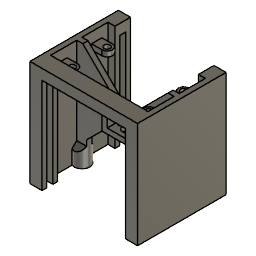
Pot_v21 (Autodesk Fusion 360 design; units mm, degrees)
Autodesk Fusion 360 part; units mm, degrees
sketch "Sketch1" plane through (0, 0, 0) normal (0, 0, 1) x (1, 0, 0)
  line L0 (0, -19.5) -> (-28, -19.5) construction
  line L1 (-28, -19.5) -> (-28, -22.5)
  line L2 (-28, -22.5) -> (-24, -22.5)
  line L3 (-28, -19.5) -> (-24, -19.5)
  line L4 (-24, -19.5) -> (-24, -16.5)
  line L5 (-24, -16.5) -> (-31, -16.5)
  line L6 (-31, -16.5) -> (-31, -25.5)
  line L7 (-31, -25.5) -> (-24, -25.5)
  line L8 (-24, -22.5) -> (-24, -25.5)
  line L9 (-24, -19.5) -> (-24, -16.5)
  line L10 (0, 0) -> (0, -19.5)
  line L11 (24, -16.5) -> (31, -16.5)
  line L12 (24, -19.5) -> (24, -16.5)
  line L13 (28, -19.5) -> (24, -19.5)
  line L14 (28, -19.5) -> (28, -22.5)
  line L15 (28, -22.5) -> (24, -22.5)
  line L16 (31, -25.5) -> (24, -25.5)
  line L17 (24, -22.5) -> (24, -25.5)
  line L18 (31, -16.5) -> (31, -25.5)
  line L19 (-28, 19.5) -> (-24, 19.5)
  line L20 (28, 19.5) -> (24, 19.5)
  line L21 (-28, 22.5) -> (-24, 22.5)
  line L22 (24, 19.5) -> (24, 16.5)
  line L23 (-31, 16.5) -> (-31, 25.5)
  line L24 (24, 19.5) -> (24, 16.5)
  line L25 (-24, 16.5) -> (-31, 16.5)
  line L26 (-24, 22.5) -> (-24, 25.5)
  line L27 (28, 22.5) -> (24, 22.5)
  line L28 (24, 16.5) -> (31, 16.5)
  line L29 (31, 16.5) -> (31, 25.5)
  line L30 (31, 25.5) -> (24, 25.5)
  line L31 (28, 19.5) -> (28, 22.5)
  line L32 (-31, 25.5) -> (-24, 25.5)
  line L33 (0, 19.5) -> (28, 19.5) construction
  line L34 (0, 0) -> (0, 19.5)
  line L35 (24, 22.5) -> (24, 25.5)
  line L36 (-24, 19.5) -> (-24, 16.5)
  line L37 (-28, 19.5) -> (-28, 22.5)
  line L38 (-31, -16.5) -> (-31, 16.5)
  line L39 (-28, 16.5) -> (-28, -16.5)
  line L40 (31, 16.5) -> (31, -16.5)
  line L41 (28, 16.5) -> (28, -16.5)
  point P0 (0, -19.5)
  point P1 (0, 19.5)
  dimension "d2" = 28
  dimension "d3" = 3
  dimension "d4" = 4
  dimension "d5" = 4
  dimension "d7" = 3
  dimension "d8" = 7
  dimension "d9" = 3
  dimension "d10" = 19.5
  dimension "d11" = 28
  dimension "d12" = 3
  dimension "d13" = 4
  dimension "d14" = 4
  dimension "d15" = 3
  dimension "d16" = 7
  dimension "d17" = 3
  dimension "d18" = 19.5
  dimension "d26" = 3
  dimension "d27" = 3
  constraint coincident P0 L0.start
  constraint horizontal L0
  constraint perpendicular L0 L1
  constraint perpendicular L1 L2
  constraint perpendicular L1 L3
  constraint perpendicular L3 L4
  constraint horizontal L5
  constraint vertical L6
  constraint horizontal L7
  constraint perpendicular L2 L8
  constraint coincident L10.start L34.start
  constraint vertical L10
  constraint symmetric L0.end L10 L13.start
  constraint symmetric L1.end L10 L14.end
  constraint symmetric L2.end L10 L15.end
  constraint symmetric L3.end L10 L12.start
  constraint symmetric L4.end L10 L11.start
  constraint symmetric L5.end L10 L11.end
  constraint symmetric L6.end L10 L16.start
  constraint symmetric L7.end L10 L16.end
  constraint coincident P1 L33.start
  constraint perpendicular L31 L33
  constraint perpendicular L27 L31
  constraint perpendicular L20 L31
  constraint perpendicular L20 L22
  constraint perpendicular L27 L35
  constraint symmetric L20.start L19.start L34
  constraint symmetric L21.start L27.start L34
  constraint symmetric L21.end L27.end L34
  constraint symmetric L20.end L19.end L34
  constraint symmetric L25.start L22.end L34
  constraint symmetric L28.end L23.start L34
  constraint symmetric L29.end L23.end L34
  constraint symmetric L30.end L26.end L34
  constraint perpendicular L33 L34
  constraint perpendicular L28 L29
  constraint perpendicular L29 L30
  constraint perpendicular L30 L35
  constraint parallel L10 L34
  constraint coincident L25 L39.start
  constraint coincident L5 L39.end
  constraint perpendicular L5 L39
  constraint coincident L28 L41.start
  constraint coincident L11 L41.end
  constraint perpendicular L28 L41
  measures "d2" distance of P0 L0.end
  measures "d3" distance of L0.end L1.end
  measures "d4" distance of L1.end L2.end
  measures "d5" distance of L0.end L3.end
  measures "d7" distance of L3.end L4.end
  measures "d8" distance of L4.end L5.end
  measures "d9" distance of L2.end L7.end
  measures "d10" distance of L10.start P0
  measures "d11" distance of P1 L20.start
  measures "d12" distance of L20.start L27.start
  measures "d13" distance of L27.end L27.start
  measures "d14" distance of L20.start L20.end
  measures "d15" distance of L20.end L22.end
  measures "d16" distance of L28.end L22.end
  measures "d17" distance of L30.end L27.end
  measures "d18" distance of P1 L10.start
  measures "d26" distance of L40 L41
  measures "d27" distance of L38 L39
extrude "Extrude1" add sketch "Sketch1" along normal blind 57.96 makes body 1 at (-31, -8.5, 19.32) makes body 2 at (31, 8.5, 19.32)
sketch "Sketch2" plane through (0, 0, 57.96) normal (0, 0, 1) x (-1, 0, 0)
  line L0 (-28, -16.5) -> (-28, 16.5)
  line L1 (-28, 16.5) -> (-24, 16.5)
  line L2 (-24, 16.5) -> (-24, 19.5)
  line L3 (-24, 19.5) -> (-28, 19.5)
  line L4 (-28, 19.5) -> (-28, 22.5)
  line L5 (-28, 22.5) -> (-24, 22.5)
  line L6 (-24, 22.5) -> (-24, 25.5)
  line L7 (-24, 25.5) -> (-31, 25.5)
  line L8 (-31, 25.5) -> (-31, -25.5)
  line L9 (-31, -25.5) -> (-24, -25.5)
  line L10 (-24, -25.5) -> (-24, -22.5)
  line L11 (-24, -22.5) -> (-28, -22.5)
  line L12 (-28, -22.5) -> (-28, -19.5)
  line L13 (-28, -19.5) -> (-24, -19.5)
  line L14 (-24, -19.5) -> (-24, -16.5)
  line L15 (-24, -16.5) -> (-28, -16.5)
  line L16 (31, -25.5) -> (-31, -25.5)
  line L17 (-31, -25.5) -> (-31, 25.5)
  line L18 (-31, 25.5) -> (31, 25.5)
  line L19 (31, 25.5) -> (31, -25.5)
  constraint horizontal L16
  constraint vertical L17
  constraint horizontal L18
  constraint vertical L19
  constraint coincident L7.end L8.start
extrude "Extrude2" add sketch "Sketch2" along normal blind 3 bodies 1 2
sketch "Sketch3" plane through (0, 0, 57.96) normal (0, 0, -1) x (1, 0, 0)
  line L0 (-24, -22.5) -> (-24, -25.5)
  line L1 (-24, -25.5) -> (24, -25.5)
  line L2 (24, -25.5) -> (24, -22.5)
  line L3 (24, -22.5) -> (28, -22.5)
  line L4 (28, -22.5) -> (28, -19.5)
  line L5 (28, -19.5) -> (24, -19.5)
  line L6 (24, -19.5) -> (24, -16.5)
  line L7 (24, -16.5) -> (28, -16.5)
  line L8 (28, -16.5) -> (28, 16.5)
  line L9 (28, 16.5) -> (24, 16.5)
  line L10 (24, 16.5) -> (24, 19.5)
  line L11 (24, 19.5) -> (28, 19.5)
  line L12 (28, 19.5) -> (28, 22.5)
  line L13 (28, 22.5) -> (24, 22.5)
  line L14 (24, 22.5) -> (24, 25.5)
  line L15 (24, 25.5) -> (-24, 25.5)
  line L16 (-24, 25.5) -> (-24, 22.5)
  line L17 (-24, 22.5) -> (-28, 22.5)
  line L18 (-28, 22.5) -> (-28, 19.5)
  line L19 (-28, 19.5) -> (-24, 19.5)
  line L20 (-24, 19.5) -> (-24, 16.5)
  line L21 (-24, 16.5) -> (-28, 16.5)
  line L22 (-28, 16.5) -> (-28, -16.5)
  line L23 (-28, -16.5) -> (-24, -16.5)
  line L24 (-24, -16.5) -> (-24, -19.5)
  line L25 (-24, -19.5) -> (-28, -19.5)
  line L26 (-28, -19.5) -> (-28, -22.5)
  line L27 (-28, -22.5) -> (-24, -22.5)
  line L28 (6.5, -5.5) -> (-6.5, -5.5)
  line L29 (-6.5, -5.5) -> (-6.5, 5.5)
  line L30 (-6.5, 5.5) -> (6.5, 5.5)
  line L31 (6.5, 5.5) -> (6.5, -5.5)
  line L32 (6.5, -5.5) -> (-6.5, 5.5) construction
  line L33 (-6.5, -5.5) -> (6.5, 5.5) construction
  line L34 (-6.5, 5.5) -> (-9.5, 5.5)
  line L35 (-9.5, 5.5) -> (-9.5, -5.5)
  line L36 (-9.5, -5.5) -> (-6.5, -5.5)
  line L37 (-6.5, -5.5) -> (-6.5, 5.5)
  line L38 (6.5, 5.5) -> (9.5, 5.5)
  line L39 (9.5, 5.5) -> (9.5, -5.5)
  line L40 (9.5, -5.5) -> (6.5, -5.5)
  line L41 (6.5, -5.5) -> (6.5, 5.5)
  line L42 (-24, -16.5) -> (24, -16.5)
  line L43 (24, 16.5) -> (-24, 16.5)
  line L44 (-9.5, 0) -> (-28, 0) construction
  line L45 (-9.5, 1.5) -> (-28, 1.5)
  line L46 (-9.5, -1.5) -> (-28, -1.5)
  line L47 (0, 0) -> (0, 5.5) construction
  line L48 (9.5, 1.5) -> (28, 1.5)
  line L49 (9.5, -1.5) -> (28, -1.5)
  line L50 (-4.5, 0) -> (4.5, 0)
  circle A0 centre (4.5, 0) radius 0.9
  circle A1 centre (-4.5, 0) radius 0.9
  line L51 (-9.5, 1.5) -> (-6.5, 1.5)
  line L52 (-9.5, -1.5) -> (-6.5, -1.5)
  line L53 (9.5, 1.5) -> (6.5, 1.5)
  line L54 (9.5, -1.5) -> (6.5, -1.5)
  line L55 (-24, 22.5) -> (-24, 19.5)
  line L56 (24, 22.5) -> (24, 19.5)
  line L57 (24, -19.5) -> (24, -22.5)
  line L58 (-24, -19.5) -> (-24, -22.5)
  circle A2 centre (-26.5, 0) radius 2.1
  line L59 (-31, 25.5) -> (-31, -25.5)
  circle A3 centre (-26.5, 0) radius 4.5
  circle A4 centre (26.5, 0) radius 4.5
  circle A5 centre (26.5, 0) radius 2.1
  circle A6 centre (22, -10) radius 3
  line L60 (22, -13) -> (28, -13)
  line L61 (22, -7) -> (28, -7)
  line L62 (0, 0) -> (0, -3) construction
  line L63 (22, -10) -> (28, -10) construction
  circle A7 centre (22, -10) radius 1.75
  line L64 (22, 13) -> (28, 13)
  circle A8 centre (22, 10) radius 3
  circle A9 centre (22, 10) radius 1.75
  line L65 (22, 7) -> (28, 7)
  circle A10 centre (-22, 10) radius 3
  circle A11 centre (-22, 10) radius 1.75
  line L66 (-22, 7) -> (-28, 7)
  line L67 (-22, 13) -> (-28, 13)
  circle A12 centre (-22, -10) radius 3
  line L68 (-22, -13) -> (-28, -13)
  line L69 (-22, -7) -> (-28, -7)
  circle A13 centre (-22, -10) radius 1.75
  circle A14 centre (0, 0) radius 3
  dimension "d30" = 13
  dimension "d31" = 11
  dimension "d32" = 3
  dimension "d33" = 3
  dimension "d41" = 1.5
  dimension "d42" = 1.5
  dimension "d43" = 9
  dimension "d44" = 1.8
  dimension "d45" = 1.8
  dimension "d61" = 4.2
  dimension "d62" = 4.5
  dimension "d75" = 6
  dimension "d76" = 6
  dimension "d77" = 10
  dimension "d78" = 3.5
  dimension "d86" = 6
  constraint horizontal L28
  constraint perpendicular L28 L29
  constraint parallel L28 L30
  constraint parallel L29 L31
  constraint coincident L32 L47.start
  constraint coincident L33 L47.start
  constraint coincident L47.start L62.start
  constraint horizontal L34
  constraint vertical L35
  constraint horizontal L36
  constraint vertical L37
  constraint horizontal L38
  constraint vertical L39
  constraint horizontal L40
  constraint vertical L41
  constraint collinear L28 L36
  constraint collinear L28 L40
  constraint coincident L23.end L24.start
  constraint coincident L6.end L7.start
  constraint coincident L9.end L10.start
  constraint coincident L20.end L21.start
  constraint midpoint L35 L44.start
  constraint midpoint L22 L44.end
  constraint coincident L35 L45.start
  constraint coincident L22 L45.end
  constraint perpendicular L22 L45
  constraint coincident L35 L46.start
  constraint coincident L22 L46.end
  constraint perpendicular L22 L46
  constraint midpoint L30 L47.end
  constraint symmetric L45.start L47 L48.start
  constraint symmetric L45.end L47 L48.end
  constraint symmetric L46.start L47 L49.start
  constraint symmetric L46.end L47 L49.end
  constraint midpoint L47.start L50
  constraint perpendicular L47 L50
  constraint coincident L50.end A0.centre
  constraint coincident L50.start A1.centre
  constraint coincident L29 L51.end
  constraint perpendicular L29 L51
  constraint coincident L29 L52.end
  constraint perpendicular L29 L52
  constraint coincident L31 L53.end
  constraint perpendicular L31 L53
  constraint coincident L31 L54.end
  constraint perpendicular L31 L54
  constraint coincident L16.end L17.start
  constraint coincident L19.end L20.start
  constraint coincident L13.end L14.start
  constraint coincident L10.end L11.start
  constraint coincident L5.end L6.start
  constraint coincident L2.end L3.start
  constraint coincident L24.end L25.start
  constraint coincident L0.start L27.end
  constraint coincident L44 A2.centre
  constraint concentric A2 A3
  constraint tangent L59 A3
  constraint symmetric L47 A2 A5
  constraint symmetric L47 A3 A4
  constraint coincident A6 L60.start
  constraint coincident L8 L60.end
  constraint perpendicular L8 L60
  constraint coincident A6 L61.start
  constraint coincident L8 L61.end
  constraint perpendicular L8 L61
  constraint perpendicular L50 L62
  constraint coincident A6.centre L63.start
  constraint coincident L8 L63.end
  constraint perpendicular L8 L63
  constraint tangent A6 L60
  constraint tangent A6 L61
  constraint concentric A6 A7
  constraint symmetric L50 A6 A8
  constraint symmetric L50 L60.start L64.start
  constraint symmetric L50 L60.end L64.end
  constraint symmetric L50 L61.start L65.start
  constraint symmetric L50 L61.end L65.end
  constraint symmetric L50 A7 A9
  constraint symmetric A6 L62 A12
  constraint symmetric L60.start L62 L68.start
  constraint symmetric L60.end L62 L68.end
  constraint symmetric L61.start L62 L69.start
  constraint symmetric L61.end L62 L69.end
  constraint symmetric L62 A7 A13
  constraint symmetric L62 L64.start L67.start
  constraint symmetric L62 L64.end L67.end
  constraint symmetric L62 A8 A10
  constraint symmetric L62 A9 A11
  constraint symmetric L62 L65.start L66.start
  constraint symmetric L62 L65.end L66.end
  measures "d30" distance of L29.end L30.end
  measures "d31" distance of L28.end L29.end
  measures "d32" distance of L29.end L34.end
  measures "d33" distance of L30.end L38.end
  measures "d41" distance of L44 L45
  measures "d42" distance of L44 L46
  measures "d43" distance of L50.start L50.end
  measures "d44" diameter of A0
  measures "d45" diameter of A1
  measures "d61" diameter of A2
  measures "d62" distance of A2.centre L59
  measures "d75" diameter of A6
  measures "d76" distance of A6.centre L63.end
  measures "d77" distance of L50 L63
  measures "d78" diameter of A7
  measures "d86" diameter of A14
extrude "Extrude3" add sketch "Sketch3" along normal blind 31 contours L22 L46 A2 | L35 L45 L46 A3 | L45 L46 A2 A3 | L22 L45 L46 A2 | L29 L35 L36 L37 L52 | L29 L35 L37 L51 L52 | L8 L49 A5 | L48 L49 A4 A5 | L39 L48 L49 A4 | L22 L45 A2 | L29 L34 L35 L37 L51 | L8 L48 L49 A5 | L31 L39 L41 L53 L54 | L31 L39 L40 L41 L54 | L8 L48 A5 | L31 L38 L39 L41 L53 bodies 1
extrude "Extrude4" add sketch "Sketch3" along normal blind 3 from surface at 28 contours L29 L35 L36 L37 L52 | L29 L35 L37 L51 L52 | L29 L34 L35 L37 L51 | L28 L29 L30 L31 L37 L41 | L31 L39 L41 L53 L54 | L31 L39 L40 L41 L54 | L31 L38 L39 L41 L53 | L50 A14 | L50 A14 | A0 | A1 bodies 1
extrude "Extrude5" cut sketch "Sketch3" against normal blind 6 contours L7 L8 L22 L23 L28 L35 L36 L39 L40 L42 L46 L49 A3 A4 A6 L60 L61 A12 L68 L69 | L22 A12 L68 L69 | A12 | L8 A6 L60 L61 | L22 L46 A2 A3 | A6 | L8 L49 A4 A5 | L46 A2 | L22 L45 A2 A3 | L8 L9 L21 L22 L30 L34 L35 L38 L39 L43 L45 L48 A3 A4 L64 A8 L65 A10 L66 L67 | L22 A10 L66 L67 | L28 L29 L30 L31 L37 L41 | L49 A5 | L8 L48 A4 A5 | L45 A2 | A10 | L48 A5 | L8 L64 A8 L65 | A8 | L50 A14 | L50 A14 | A0 | A1 | A7 | A9 | A11 | A13 bodies 1
extrude "Extrude6" cut sketch "Sketch3" along normal blind 32 contours A0 | A1 bodies 1
extrude "Extrude7" cut sketch "Sketch3" along normal blind 15 and the other way blind 5 contours L29 L35 L36 L37 L52 | L29 L34 L35 L37 L51 | L31 L39 L40 L41 L54 | L31 L38 L39 L41 L53 bodies 1
chamfer "Chamfer2" distance 18 distance2 18 2 edges at (-6.5, 0, 60.96) (6.5, 0, 60.96) measured on face at (-9.3333, -22.5, 60.96) measured on face at (-9.3333, -22.5, 60.96) tangent chain off on bodies 1
chamfer "Chamfer3" distance 4 distance2 4 4 edges at (8, 5.5, 42.96) (8, -5.5, 42.96) (-8, -5.5, 42.96) (-8, 5.5, 42.96) measured on face at (2.1667, 5.5, 27.96) measured on face at (-2.1667, -5.5, 27.96) measured on face at (-2.1667, -5.5, 27.96) measured on face at (2.1667, 5.5, 27.96) tangent chain off on bodies 1
extrude "Extrude8" add sketch "Sketch3" along normal blind 3 contours L0 L1 L2 L6 L24 L42 L57 L58 | L25 L26 L27 L58 | L3 L4 L5 L57 | L10 L14 L15 L16 L20 L43 L55 L56 | L17 L18 L19 L55 | L11 L12 L13 L56 bodies 1
chamfer "Chamfer4" distance 18.5 angle 45 2 edges at (-28, 0, 26.96) (28, 0, 26.96) tangent chain off on bodies 1
extrude "Extrude9" add sketch "Sketch3" along normal blind 7.96 from surface at 50 contours L22 L46 A2 A3 | L45 L46 A2 A3 | L8 L49 A4 A5 | L22 L45 L46 A2 | L46 A2 | L22 L45 A2 A3 | L48 L49 A4 A5 | L8 L48 L49 A5 | L49 A5 | L8 L48 A4 A5 | L45 A2 | L48 A5 bodies 1
delete_face "DeleteFace1" 1 faces at (27.9798, -1.5, 5.3067) on bodies 1
delete_face "DeleteFace2" 1 faces at (27.9967, 1.4731, 2.6533) on bodies 1
delete_face "DeleteFace3" 1 faces at (-27.9798, -1.5, 5.3067) on bodies 1
delete_face "DeleteFace4" 1 faces at (-27.9731, 1.4967, 2.6533) on bodies 1
extrude "Extrude10" add sketch "Sketch3" along normal blind 57.96 contours L45 L46 A2 A3 | L22 L45 L46 A2 | L48 L49 A4 A5 | L8 L48 L49 A5 bodies 1
chamfer "Chamfer5" distance 2.9999 angle 45 4 edges at (25.1135, -1.5, 7.96) (-25.1135, -1.5, 7.96) (-25.1135, 1.5, 7.96) (25.1135, 1.5, 7.96) tangent chain off on bodies 1
hole "Hole1" at (26.5, 0, 0) direction (0, 0, 1) diameter 4.2 depth 6 tip angle 180 bodies 1
hole "Hole2" at (-26.5, 0, 0) direction (0, 0, 1) diameter 4.2 depth 6 tip angle 180 bodies 1
extrude "Extrude11" add sketch "Sketch3" along normal blind 3 from surface at 3 contours L22 A12 L68 L69 | A12 | L8 A6 L60 L61 | A6 | L22 A10 L66 L67 | A10 | L8 L64 A8 L65 | A8 bodies 1
extrude "Extrude13" cut sketch "Sketch3" along normal blind 43 contours L50 A14 | L50 A14 bodies 1
sketch "Sketch4" plane through (0, 0, 54.96) normal (0, 0, -1) x (1, 0, 0)
  line L0 (-24, -19.5) -> (-28, -19.5)
  line L1 (-28, -19.5) -> (-28, -22.5)
  line L2 (-28, -22.5) -> (-24, -22.5)
  line L3 (-24, -22.5) -> (-24, -25.5)
  line L4 (-24, -25.5) -> (24, -25.5)
  line L5 (24, -25.5) -> (24, -22.5)
  line L6 (24, -22.5) -> (28, -22.5)
  line L7 (28, -22.5) -> (28, -19.5)
  line L8 (28, -19.5) -> (24, -19.5)
  line L9 (24, -19.5) -> (24, -16.5)
  line L10 (24, -16.5) -> (-24, -16.5)
  line L11 (-24, -16.5) -> (-24, -19.5)
  line L12 (24, -19.5) -> (24, -22.5)
  line L13 (-24, -19.5) -> (-24, -22.5)
  constraint coincident L8.end L9.start
  constraint coincident L5.end L6.start
  constraint coincident L0.start L11.end
  constraint coincident L2.end L3.start
extrude "Extrude14" cut sketch "Sketch4" against normal blind 14 contours L3 L4 L5 L9 L10 L11 L12 L13 bodies 1
move_face "OffsetFaces1" offset -0.2 3 faces at (-26.6667, 19.5, 18.32) (-28, 21.5, 18.32) (-26.6667, 22.5, 18.32) on bodies 1
move_face "OffsetFaces2" offset -0.2 3 faces at (-26.6667, -19.5, 18.32) (-28, -20.5, 18.32) (-26.6667, -22.5, 18.32) on bodies 1
move_face "OffsetFaces3" offset -0.2 3 faces at (26.6667, -22.5, 18.32) (28, -21.5, 36.64) (26.6667, -19.5, 18.32) on bodies 1
move_face "OffsetFaces4" offset -0.2 3 faces at (26.6667, 19.5, 18.32) (28, 21.5, 18.32) (25.3333, 22.5, 36.64) on bodies 1
equation "d2 = ( 56 / 2 ) * 1 mm"
equation "d11 = ( 56 / 2 ) * 1 mm"
equation "d24 = 54.96 mm + 3 mm"
equation "d48 = 25.00 mm - 10 mm"
